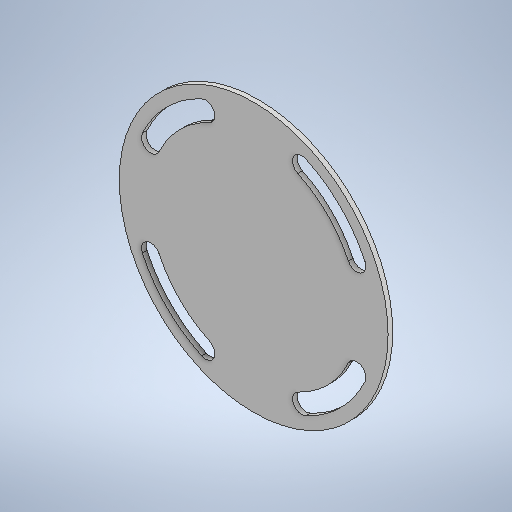
# Autodesk Inventor part: MSC 126 flange frame
Saved by Autodesk Inventor 2025 (Build 290162010, 162A)
## iProperties
Created: 2024-07-01
Part Number: MSC 126 flange frame
Material: Stainless Steel
Document SubType Name: Sheet Metal
Designer: pokla
Density: 8 g/cm^3
Sheet Metal Rule: AISI304 2mm Die16
Appearance: Default
Author: pokla
Autodesk Inventor part; units mm, degrees
ref_plane "YZ Plane" through (0, 0, 0) normal (1, 0, 0) x (0, 1, 0)
ref_plane "XZ Plane" through (0, 0, 0) normal (0, 1, 0) x (-1, 0, 0)
ref_plane "XY Plane" through (0, 0, 0) normal (0, 0, 1) x (1, 0, 0)
sketch "Sketch1" plane through (0, 0, 0) normal (0, 1, 0) x (-1, 0, 0)
  circle A0 centre (0, 0) radius 87.5
  dimension "d0" = 175
  measures "d0" diameter of A0
extrude "Plate1" add sketch "Sketch1" along normal blind 3
sketch "Sketch2" plane through (0, 3, 0) normal (0, 1, 0) x (1, 0, 0)
  line L0 (-40, -40) -> (40, -40) construction
  line L1 (40, -40) -> (40, 40) construction
  line L2 (40, 40) -> (-40, 40) construction
  line L3 (-40, 40) -> (-40, -40) construction
  line L4 (-40, -40) -> (40, 40) construction
  circle A0 centre (0, 0) radius 87.5 projected
  circle A1 centre (0, 0) radius 74 construction
  circle A2 centre (-67.0668, -31.2738) radius 6
  line L5 (-67.0668, -31.2738) -> (0, 0) construction
  circle A3 centre (-31.2738, -67.0668) radius 6
  line L6 (-31.2738, -67.0668) -> (0, 0) construction
  arc A4 (-72.5046, -33.8095) -> (-33.8095, -72.5046) centre (0, 0) ccw
  arc A5 (-61.6289, -28.738) -> (-28.738, -61.6289) centre (0, 0) ccw
  point P0 (-61.6289, -28.738)
  point P1 (-28.738, -61.6289)
  dimension "d7" = 12
  dimension "d9" = 12
  dimension "d2" = 80
  dimension "d3" = 80
  dimension "d16" = 40
  dimension "d17" = 20
  dimension "d18" = 13.5
  constraints: 14 end point, 6 point on circle, 4 coincident, 3 centre point, 2 parallel, 2 point on line, 1 horizontal, 1 midpoint, 1 perpendicular, 8 other
  measures "d2" distance of L2.end L1.end
  measures "d3" distance of L0.end L1.end
  measures "d16" angle of L5 L6
  measures "d17" angle of L6 L4
  measures "d18" radial gap between concentric circles of A0 A1
extrude "Extrusion1" cut sketch "Sketch2" against normal through all contours A2 | A2 A5 A3 A4 | A3
pattern_circular "Circular Pattern1" count 4 over 360 about axis through (0, -10, 0) along (0, 1, 0) of "Extrusion1"
equation "\"d9\" = d7"
equation "\"BendReliefWidth\" = Thickness"
equation "\"BendReliefDepth\" = 0.5 * Thickness"
equation "\"CornerReliefSize\" = 4 * Thickness"
equation "\"MinimumRemnant\" = 2 * Thickness"
equation "\"TransitionRadius\" = BendRadius"
equation "\"JacobiRadiusSize\" = BendRadius"
equation "\"GapSize\" = Thickness"
body "Solid1"
